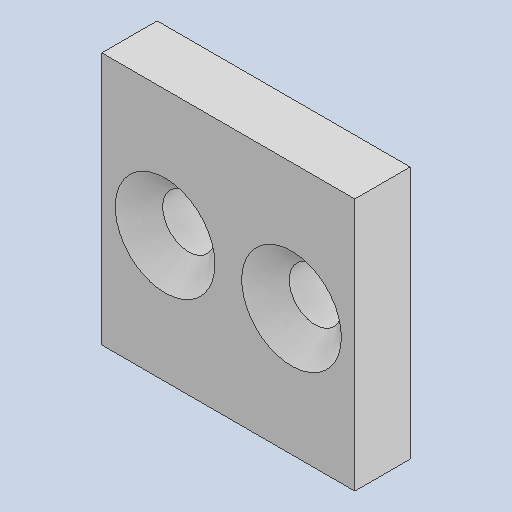
# Autodesk Inventor part: grampo_trava
Saved by Autodesk Inventor 2022.2 (Build 262287010, 287A)
## iProperties
Created: 2022-03-09
Part Number: grampo_trava
Material: Genérico
Document SubType Name: Modeling
Designer: 19710060
Density: 1 g/cm^3
Appearance: Padrão
Author: 19710060
Autodesk Inventor part; units mm, degrees
ref_plane "YZ Plane" through (0, 0, 0) normal (1, 0, 0) x (0, 1, 0)
ref_plane "XZ Plane" through (0, 0, 0) normal (0, 1, 0) x (-1, 0, 0)
ref_plane "XY Plane" through (0, 0, 0) normal (0, 0, 1) x (1, 0, 0)
sketch "Esboço1" plane through (0, 0, 0) normal (0, 0, 1) x (1, 0, 0)
  line L0 (0, 0) -> (32, 0)
  line L1 (32, 0) -> (32, 32)
  line L2 (32, 32) -> (0, 32)
  line L3 (0, 32) -> (0, 0)
  line L4 (8, 16) -> (24, 16)
  dimension "d0" = 32
  dimension "d1" = 32
  dimension "d3" = 16
  constraints: 10 end point, 2 parallel, 1 horizontal, 1 perpendicular
  measures "d0" distance of L2.end L1.end
  measures "d1" distance of L1.end L0.end
  measures "d3" distance of L4.start L4.end
extrude "Extrusão1" add sketch "Esboço1" against normal blind 7
hole "Furo1" at (8, 16, 0) at (24, 16, 0) direction (0, 0, -1) diameter 6.6 end through all countersink diameter 12.6 countersink angle 90
